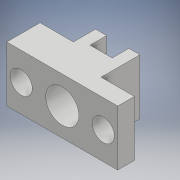
# Autodesk Inventor part: P3-10
Saved by Autodesk Inventor 2017 (Build 210142000, 142)
## iProperties
Created: 2017-02-12
Part Number: P3-10
Material: Generic
Document SubType Name: Modeling
Designer: Schaffel
Density: 1 g/cm^3
Appearance: Default
Author: Schaffel
Autodesk Inventor part; units mm, degrees
ref_plane "YZ Plane" through (0, 0, 0) normal (1, 0, 0) x (0, 1, 0)
ref_plane "XZ Plane" through (0, 0, 0) normal (0, 1, 0) x (-1, 0, 0)
ref_plane "XY Plane" through (0, 0, 0) normal (0, 0, 1) x (1, 0, 0)
sketch "Sketch1" plane through (0, 0, 0) normal (0, 0, 1) x (1, 0, 0)
  line L0 (0, 0) -> (100, 0)
  line L1 (100, 0) -> (100, 15)
  line L2 (100, 15) -> (70, 15)
  line L3 (70, 15) -> (70, 50)
  line L4 (70, 50) -> (30, 50)
  line L5 (30, 50) -> (30, 30)
  line L6 (30, 30) -> (0, 30)
  line L7 (0, 30) -> (0, 0)
  dimension "d0" = 100
  dimension "d1" = 15
  dimension "d2" = 30
  dimension "d3" = 35
  constraints: 16 end point, 6 perpendicular, 1 horizontal, 1 parallel
  measures "d0" distance of L0.start L0.end
  measures "d1" distance of L0.end L1.end
  measures "d2" distance of L1.end L2.end
  measures "d3" distance of L2.end L3.end
extrude "Extrusion1" add sketch "Sketch1" along normal blind 50
sketch "Sketch2" plane through (0, 0, 0) normal (0, -1, 0) x (1, 0, 0)
  circle A0 centre (13, 25) radius 10
  circle A1 centre (87, 25) radius 10
  circle A2 centre (50, 25) radius 15
  point P0 (0, 0)
  constraints: 3 centre point
extrude "Extrusion2" cut sketch "Sketch2" against normal blind 50
sketch "Sketch3" plane through (0, 0, 50) normal (0, 0, 1) x (1, 0, 0)
  line L0 (70, 50) -> (30, 50) projected
  line L1 (40, 50) -> (40, 35)
  line L2 (40, 35) -> (60, 35)
  line L3 (60, 35) -> (60, 50)
  line L4 (40, 50) -> (60, 50)
  line L5 (35, 50) -> (65, 50) projected
  point P0 (0, 0)
  constraints: 8 end point, 2 perpendicular, 2 point on line, 1 collinear
extrude "Extrusion3" cut sketch "Sketch3" against normal blind 15
body "Solid1"
